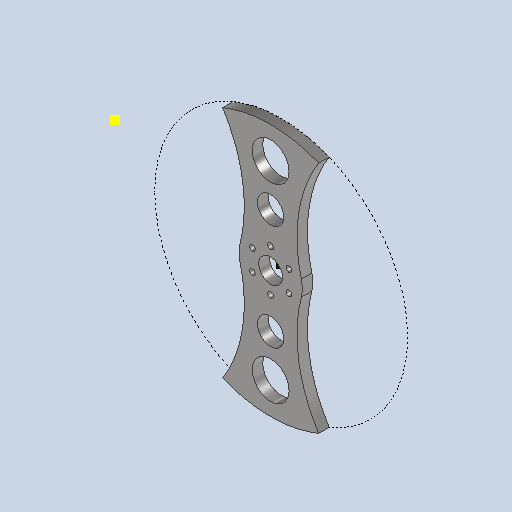
# Autodesk Inventor part: Blade (Bar)
Saved by Autodesk Inventor 2023.1 (Build 271208000, 208)
## iProperties
Created: 2022-06-12
Part Number: Blade (Bar)
Material: Stainless Steel
Document SubType Name: Modeling
Designer: Nathan Cai
Density: 8 g/cm^3
Appearance: Semi-Polished
Mass: 224.322 g
Surface Area: 136.703 cm^2
Volume: 28.0402 cm^3
Author: Nathan Cai
Autodesk Inventor part; units mm, degrees
ref_plane "YZ Plane" through (0, 0, 0) normal (1, 0, 0) x (0, 1, 0)
ref_plane "XZ Plane" through (0, 0, 0) normal (0, 1, 0) x (-1, 0, 0)
ref_plane "XY Plane" through (0, 0, 0) normal (0, 0, 1) x (1, 0, 0)
sketch "Sketch1" plane through (0, 0, 0) normal (0, 0, 1) x (1, 0, 0)
  circle A0 centre (0, 0) radius 7.1437
  line L0 (0, 0) -> (0, 12.7) construction
  circle A1 centre (0, 12.7) radius 1.7526
  circle A2 centre (-10.9985, 6.35) radius 1.7526
  circle A3 centre (-10.9985, -6.35) radius 1.7526
  circle A4 centre (0, -12.7) radius 1.7526
  circle A5 centre (10.9985, -6.35) radius 1.7526
  circle A6 centre (10.9985, 6.35) radius 1.7526
  circle A7 centre (0, 0) radius 76.2 construction
  line L1 (-15.875, -74.528) -> (15.875, -74.528) construction
  line L2 (15.875, -74.528) -> (15.875, 74.528) construction
  line L3 (15.875, 74.528) -> (-15.875, 74.528) construction
  line L4 (-15.875, 74.528) -> (-15.875, -74.528) construction
  line L5 (-15.875, -74.528) -> (15.875, 74.528) construction
  line L6 (15.875, -74.528) -> (-15.875, 74.528) construction
  line L7 (0, 76.2) -> (0, -76.2) construction
  line L8 (0, 0) -> (28.9333, 70.4933) construction
  circle A8 centre (0, 0) radius 66.675 construction
  circle A9 centre (0, 0) radius 19.05
  arc A10 (28.9333, 70.4933) -> (18.4648, 4.6853) centre (100.1873, 25.4218) ccw
  line L9 (28.9333, 70.4933) -> (23.7514, 62.3011) construction
  arc A11 (-18.4648, 4.6853) -> (-28.9333, 70.4933) centre (-100.1873, 25.4218) ccw
  arc A12 (28.9333, 70.4933) -> (-28.9333, 70.4933) centre (0, 0) ccw
  line L10 (-15.875, 0) -> (15.875, 0) construction
  circle A13 centre (0, 57.15) radius 11.1125
  circle A14 centre (0, 31.75) radius 7.9375
  arc A15 (18.4648, -4.6853) -> (28.9333, -70.4933) centre (100.1873, -25.4218) ccw
  arc A16 (-28.9333, -70.4933) -> (-18.4648, -4.6853) centre (-100.1873, -25.4218) ccw
  arc A17 (-28.9333, -70.4933) -> (28.9333, -70.4933) centre (0, 0) ccw
  circle A18 centre (0, -57.15) radius 11.1125
  circle A19 centre (0, -31.75) radius 7.9375
  point P0 (0, 74.528)
  point P1 (0, -66.675)
  point P2 (-17.412, -7.7282)
  point P3 (17.412, -7.7282)
  point P4 (-18.4648, -4.6853)
  point P5 (18.4648, -4.6853)
  dimension "d0" = 14.2875
  dimension "d1" = 12.7
  dimension "d2" = 3.5052
  dimension "d5" = 360
  dimension "d7" = 152.4
  dimension "d8" = 31.75
  dimension "d9" = 9.525
  dimension "d10" = 38.1
  dimension "d11" = 10
  dimension "d12" = 22.225
  dimension "d13" = 57.15
  dimension "d14" = 15.875
  dimension "d15" = 31.75
  constraints: 23 point on circle, 22 end point, 20 centre point, 11 symmetric about line, 7 midpoint, 4 coincident, 3 point on line, 3 tangent, 2 parallel, 2 perpendicular, 1 concentric, 1 horizontal, 1 vertical, 19 other
  measures "d0" diameter of A0
  measures "d1" distance of L0.start L0.end
  measures "d2" diameter of A1
  measures "d7" diameter of A7
  measures "d8" distance of L3.end L2.end
  measures "d9" radial gap between concentric circles of A7 A8
  measures "d10" diameter of A9
  measures "d11" angle of L9 L8
  measures "d12" diameter of A13
  measures "d13" distance of point (0, 0) A13.centre
  measures "d14" diameter of A14
  measures "d15" distance of point (0, 0) A14.centre
extrude "Extrusion1" add sketch "Sketch1" along normal blind 6.35
sketch "Sketch2" plane through (0, 0, 6.35) normal (0, 0, 1) x (1, 0, 0)
  arc A0 (28.9333, 70.4933) -> (-28.9333, 70.4933) centre (0, 0) ccw projected
  line L0 (28.9333, 70.4933) -> (-4.1978, 84.0916)
  point P0 (0, 0)
  constraints: 2 end point, 1 tangent
sketch "Sketch3" plane through (0, 0, 0) normal (0, 0, -1) x (-1, 0, 0)
  arc A0 (28.9333, 70.4933) -> (18.4648, 4.6853) centre (100.1873, 25.4218) ccw projected
  circle A1 centre (0, 0) radius 76.2 construction
  constraints: 1 coincident, 3 other
body "Solid1"
